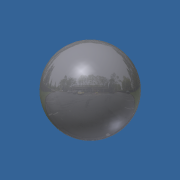
# Autodesk Inventor part: ball_bearing
Saved by Autodesk Inventor 2011 (Build 150239000, 239)
## iProperties
Created: 2011-01-09
Part Number: ball_bearing
Material: Stainless Steel
Document SubType Name: Modeling
Designer: Antonella Wilby
Mass: 16.9259 g
Surface Area: 7.9173 cm^2
Volume: 2.09479 cm^3
Density: 8.08 g/cm^3
Author: Antonella Wilby
Autodesk Inventor part; units mm, degrees
ref_plane "YZ Plane" through (0, 0, 0) normal (1, 0, 0) x (0, 1, 0)
ref_plane "XZ Plane" through (0, 0, 0) normal (0, 1, 0) x (-1, 0, 0)
ref_plane "XY Plane" through (0, 0, 0) normal (0, 0, 1) x (1, 0, 0)
sketch "Sketch1" plane through (0, 0, 0) normal (0, 0, 1) x (1, 0, 0)
  line L0 (-9.525, 0) -> (1.5875, 0) projected
  line L1 (0, -11.1125) -> (0, 11.1125) projected
  arc A0 (0, 7.9375) -> (0, -7.9375) centre (0, 0) ccw
  line L2 (0, 7.9375) -> (0, -7.9375)
  dimension "d0" = 7.9375
  constraints: 2 end point, 2 point on circle, 2 point on line, 1 centre point, 1 coincident
  measures "d0" radius of A0
revolve "Revolution1" add sketch "Sketch1" angle 360 about axis through (0, -10, 0) along (0, 1, 0)
body "Solid1"
